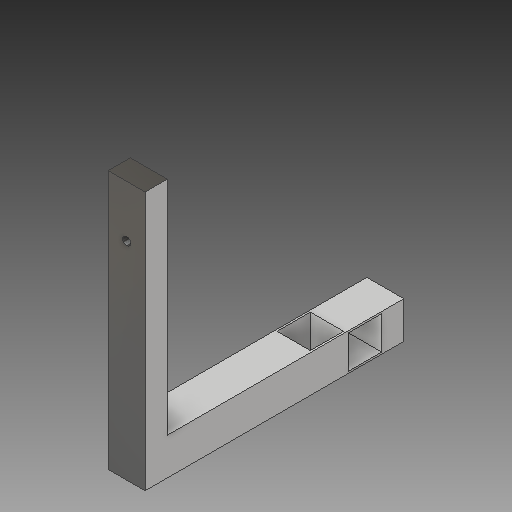
# Autodesk Inventor part: brazo
Saved by Autodesk Inventor 2019 (Build 230136000, 136)
## iProperties
Created: 2019-08-08
Part Number: brazo
Material: Generic
Document SubType Name: Modeling
Designer: felix
Density: 1 g/cm^3
Appearance: Default
Mass: 1119.69 g
Surface Area: 1337.42 cm^2
Volume: 1119.69 cm^3
Author: felix
Autodesk Inventor part; units mm, degrees
ref_plane "YZ Plane" through (0, 0, 0) normal (1, 0, 0) x (0, 1, 0)
ref_plane "XZ Plane" through (0, 0, 0) normal (0, 1, 0) x (-1, 0, 0)
ref_plane "XY Plane" through (0, 0, 0) normal (0, 0, 1) x (1, 0, 0)
sketch "Sketch1" plane through (0, 0, 0) normal (0, 0, 1) x (1, 0, 0)
  line L0 (-25, 25) -> (25, 25)
  line L1 (25, 25) -> (25, -25)
  line L2 (25, -25) -> (-25, -25)
  line L3 (-25, -25) -> (-25, 25)
  point P0 (0, 0)
  dimension "d0" = 50
  dimension "d1" = 25
  dimension "d2" = 25
  dimension "d3" = 25
  constraints: 8 end point, 2 parallel, 1 horizontal, 1 perpendicular
  measures "d0" distance of L2.end L0.start
  measures "d1" horizontal distance of L0.end point (0, 0)
  measures "d2" horizontal distance of L1.end point (0, 0)
  measures "d3" horizontal distance of L0.start point (0, 0)
extrude "Extrusion1" add sketch "Sketch1" along normal blind 350
sketch "Sketch2" plane through (-25, 25, 0) normal (0, 1, 0) x (1, 0, 0)
  line L0 (50, -350) -> (0, -350) projected
  line L1 (50, 0) -> (50, -350) projected
  line L2 (0, -350) -> (50, -350)
  line L3 (50, -350) -> (50, -320)
  line L4 (50, -320) -> (0, -320)
  line L5 (0, -320) -> (0, -350)
  point P0 (25, 0)
  dimension "d6" = 30
  constraints: 8 end point, 2 parallel, 1 horizontal, 1 perpendicular, 1 point on line
  measures "d6" distance of L3.end L2.end
extrude "Extrusion2" add sketch "Sketch2" along normal blind 300
sketch "Sketch3" plane through (0, 0, 350) normal (0, 0, 1) x (1, 0, 0)
  line L0 (-25, 325) -> (25, 325) projected
  line L1 (25, -25) -> (25, 325) projected
  point P0 (0, 0)
  point P1 (0, 255)
  dimension "d9" = 70
  dimension "d10" = 25
  measures "d9" distance from line of L0 point (0, 255)
  measures "d10" distance from line of L1 point (0, 255)
hole "Hole1" at (0, 255, 350) direction (0, 0, -1) diameter 10.917 end through all thread size "M12x1" class "6H" standard "ANSI Metric M Profile"
sketch "Sketch6" plane through (25, -25, 0) normal (1, 0, 0) x (0, 0, -1)
  line L0 (-75, 2.5) -> (-30, 2.5)
  line L1 (-30, 2.5) -> (-30, 47.5)
  line L2 (-30, 47.5) -> (-75, 47.5)
  line L3 (-75, 47.5) -> (-75, 2.5)
  line L4 (0, 50) -> (0, 0) projected
  line L5 (0, 0) -> (-350, 0) projected
  point P0 (0, 25)
  dimension "d36" = 45
  dimension "d37" = 45
  dimension "d38" = 30
  dimension "d39" = 2.5
  constraints: 8 end point, 2 parallel, 1 horizontal, 1 perpendicular
  measures "d36" distance of L2.end L1.end
  measures "d37" distance of L1.end L0.end
  measures "d38" distance between parallel lines of L1 L4
  measures "d39" distance between parallel lines of L5 L0
extrude "Extrusion3" cut sketch "Sketch6" against normal blind 50
sketch "Sketch7" plane through (-25, -25, 0) normal (0, -1, 0) x (1, 0, 0)
  line L0 (50, 0) -> (0, 0) projected
  line L1 (50, 0) -> (50, 350) projected
  point P0 (25, 0)
  point P1 (25, 102)
  dimension "d42" = 102
  dimension "d43" = 25
  measures "d42" distance from line of L0 point (25, 102)
  measures "d43" distance from line of L1 point (25, 102)
hole "Hole4" at (0, -25, 102) direction (0, 1, 0) diameter 11.835 end through all thread size "M14x2" class "6H" standard "ANSI Metric M Profile"
sketch "Sketch8" plane through (-25, -25, 0) normal (0, -1, 0) x (1, 0, 0)
  line L0 (2.5, 124) -> (47.5, 124)
  line L1 (47.5, 124) -> (47.5, 79)
  line L2 (47.5, 79) -> (2.5, 79)
  line L3 (2.5, 79) -> (2.5, 124)
  line L4 (50, 0) -> (0, 0) projected
  line L5 (0, 0) -> (0, 350) projected
  point P0 (25, 0)
  dimension "d51" = 45
  dimension "d52" = 45
  dimension "d53" = 79
  dimension "d54" = 2.5
  constraints: 8 end point, 2 parallel, 1 horizontal, 1 perpendicular
  measures "d51" distance of L1.end L2.end
  measures "d52" distance of L0.end L1.end
  measures "d53" distance between parallel lines of L4 L2
  measures "d54" distance between parallel lines of L5 L3
extrude "Extrusion4" cut sketch "Sketch8" against normal blind 50
sketch "Sketch9" plane through (25, -25, 0) normal (1, 0, 0) x (0, 0, -1)
  line L0 (0, 50) -> (0, 0) projected
  line L1 (0, 0) -> (-350, 0) projected
  point P0 (0, 25)
  point P1 (-52.5, 25)
  dimension "d57" = 52.5
  dimension "d58" = 25
  measures "d57" distance from line of L0 point (-52.5, 25)
  measures "d58" distance from line of L1 point (-52.5, 25)
hole "Hole5" at (25, 0, 52.5) direction (-1, 0, 0) diameter 11.835 end through all thread size "M14x2" class "6H" standard "ANSI Metric M Profile"
body "Solid1"
